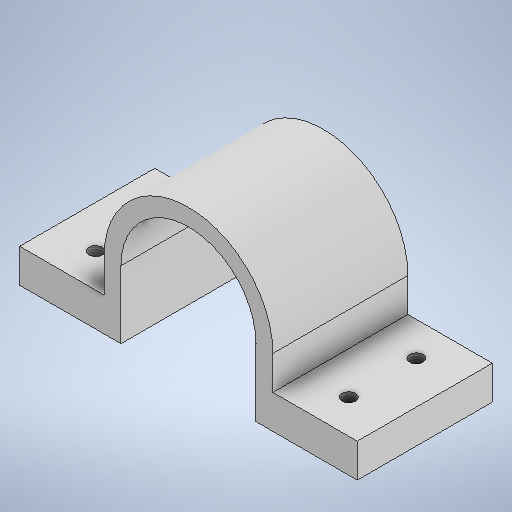
# Autodesk Inventor part: U-bracket
Saved by Autodesk Inventor 2025.3 (Build 293356030, 356C)
## iProperties
Created: 2026-06-26
Part Number: U-bracket
Material: Generic
Document SubType Name: Modeling
Designer: user
Density: 1 g/cm^3
Appearance: Default
Author: user
Autodesk Inventor part; units mm, degrees
ref_plane "YZ Plane" through (0, 0, 0) normal (1, 0, 0) x (0, 1, 0)
ref_plane "XZ Plane" through (0, 0, 0) normal (0, 1, 0) x (-1, 0, 0)
ref_plane "XY Plane" through (0, 0, 0) normal (0, 0, 1) x (1, 0, 0)
sketch "Sketch1" plane through (0, 0, 0) normal (0, 0, 1) x (1, 0, 0)
  arc A0 (20, 20) -> (-20, 20) centre (0, 20) ccw
  line L0 (50, 0) -> (50, 10)
  line L1 (-50, 10) -> (-50, 0)
  line L2 (50, 10) -> (25, 10)
  line L3 (-25, 10) -> (-50, 10)
  line L4 (20, 20) -> (20, 0)
  line L5 (-20, 20) -> (-20, 0)
  line L6 (25, 20) -> (25, 10)
  line L7 (-25, 20) -> (-25, 10)
  arc A1 (25, 20) -> (-25, 20) centre (0, 20) ccw
  line L8 (-50, 0) -> (-20, 0)
  line L9 (20, 0) -> (50, 0)
  point P0 (0, 0)
  point P1 (0, 40)
  dimension "d1" = 10
  dimension "d4" = 50
  dimension "d5" = 25
  dimension "d6" = 25
  dimension "d7" = 50
  dimension "d22" = 25
  dimension "d23" = 20
  dimension "d24" = 20
  dimension "d25" = 40
  dimension "d26" = 10
  constraints: 20 end point, 7 parallel, 6 point on circle, 4 perpendicular, 4 tangent, 2 centre point, 2 horizontal, 1 coincident
  measures "d1" distance of L0.end L0.start
  measures "d4" horizontal distance of L0.end A0.centre
  measures "d5" distance of L0.end L2.end
  measures "d6" distance of L3.start L1.start
  measures "d7" distance from line of L1 A0.centre
  measures "d22" radius of A1
  measures "d23" radius of A0
  measures "d24" distance of L4.end point (0, 0)
  measures "d25" distance of point (0, 0) point (0, 40)
  measures "d26" distance from line of point (0, 0) L3
extrude "Extrusion1" add sketch "Sketch1" along normal blind 40
sketch "Sketch2" plane through (25, 10, 0) normal (0, 1, 0) x (1, 0, 0)
  point P0 (-25, 0)
sketch "Sketch3" plane through (25, 10, 0) normal (0, 1, 0) x (1, 0, 0)
  line L0 (25, 0) -> (0, 0) construction
  line L1 (12.5, 0) -> (12.5, -40) construction
  line L2 (25, -40) -> (0, -40) construction
  line L3 (25, 0) -> (25, -40) construction
  line L4 (25, -20) -> (-75, -20) construction
  line L5 (-75, 0) -> (-75, -40) construction
  line L6 (-50, 0) -> (-75, 0) construction
  line L7 (-62.5, 0) -> (-62.5, -40) construction
  line L8 (-50, -40) -> (-75, -40) construction
  line L9 (-77.5, -10) -> (32.5, -10) construction
  line L10 (-75, -30) -> (25, -30) construction
  circle A0 centre (12.5, -10) radius 2
  circle A1 centre (12.5, -30) radius 2
  circle A2 centre (-62.5, -10) radius 2
  circle A3 centre (-62.5, -30) radius 2
  point P0 (-25, 0)
  dimension "d8" = 4
  dimension "d9" = 4
  dimension "d10" = 4
  dimension "d11" = 4
  constraints: 10 end point, 10 point on line, 6 midpoint, 4 centre point, 1 horizontal, 1 perpendicular
  measures "d8" diameter of A0
  measures "d9" diameter of A1
  measures "d10" diameter of A2
  measures "d11" diameter of A3
extrude "Extrusion2" cut sketch "Sketch3" against normal blind 10
thread "Thread1" size "M4x0.7" class "6H" standard "ISO Metric profile" length 150
thread "Thread2" size "M4x0.7" class "6H" standard "ISO Metric profile" length 150
thread "Thread3" size "M4x0.7" class "6H" standard "ISO Metric profile" length 150
thread "Thread4" size "M4x0.7" class "6H" standard "ISO Metric profile" length 150
body "Solid1"
